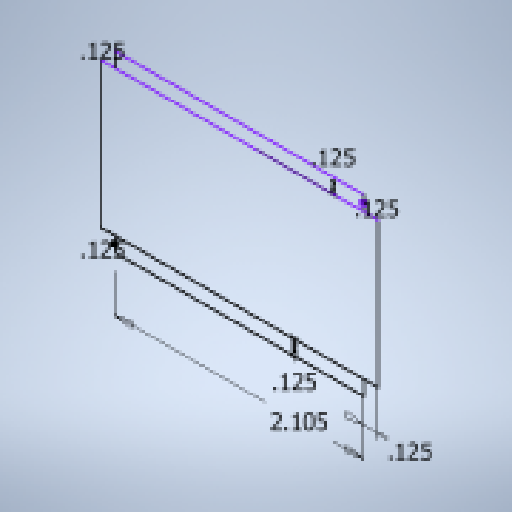
# Autodesk Inventor part: servo long side
Saved by Autodesk Inventor 2023 (Build 270158000, 158)
## iProperties
Created: 2023-11-14
Part Number: servo long side
Material: Generic
Document SubType Name: Modeling
Designer: Nate
Density: 1 g/cm^3
Appearance: Default
Author: Nate
Autodesk Inventor part; units mm, degrees
ref_plane "YZ Plane" through (0, 0, 0) normal (1, 0, 0) x (0, 1, 0)
ref_plane "XZ Plane" through (0, 0, 0) normal (0, 1, 0) x (-1, 0, 0)
ref_plane "XY Plane" through (0, 0, 0) normal (0, 0, 1) x (1, 0, 0)
sketch "Sketch1" plane through (0, 0, 0) normal (0, 0, 1) x (1, 0, 0)
  line L0 (0, 0) -> (59.817, 0)
  line L1 (59.817, 0) -> (59.817, 20.066)
  line L2 (59.817, 20.066) -> (0, 20.066)
  line L3 (0, 20.066) -> (0, 0)
  line L4 (3.175, 0) -> (56.642, 0)
  line L5 (56.642, 0) -> (56.642, -3.175)
  line L6 (56.642, -3.175) -> (3.175, -3.175)
  line L7 (3.175, -3.175) -> (3.175, 0)
  line L8 (3.175, 20.066) -> (56.642, 20.066)
  line L9 (56.642, 20.066) -> (56.642, 23.241)
  line L10 (56.642, 23.241) -> (3.175, 23.241)
  line L11 (3.175, 23.241) -> (3.175, 20.066)
  point P0 (3.175, -1.5875)
  point P1 (56.642, 21.6535)
  dimension "d0" = 3.175
  dimension "d1" = 3.175
  dimension "d2" = 3.175
  dimension "d4" = 53.467
  dimension "d5" = 3.175
  dimension "d6" = 3.175
  dimension "d7" = 3.175
  dimension "d8" = 20.066
  constraints: 24 end point, 6 parallel, 3 horizontal, 3 perpendicular, 2 midpoint, 2 point on line
  measures "d0" distance between parallel lines of L0 L6
  measures "d1" distance between parallel lines of L3 L7
  measures "d2" distance between parallel lines of L1 L5
  measures "d4" distance from line of L5 point (3.175, -1.588)
  measures "d5" distance between parallel lines of L3 L11
  measures "d6" distance between parallel lines of L10 L2
  measures "d7" distance from line of L1 point (56.642, 21.654)
  measures "d8" distance between parallel lines of L2 L0
extrude "Extrusion1" add sketch "Sketch1" along normal blind 3.175
body "Solid1"
